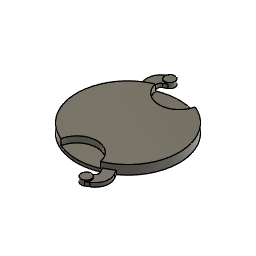
Deckbox - Key (Autodesk Fusion 360 design; units mm, degrees)
Autodesk Fusion 360 part; units mm, degrees
sketch "Sketch1" plane through (0, 0, 0) normal (0, 1, 0) x (1, 0, 0)
  circle A0 centre (0, 0) radius 25.4
  line L0 (19.5918, -28.934) -> (-15.2617, 31.434)
  line L1 (-19.5918, 28.934) -> (15.2617, -31.434)
  line L2 (0, -25.4) -> (0, 25.4) construction
  line L3 (0, 0) -> (25.4, 0) construction
  line L4 (-19.5918, 28.934) -> (-15.2617, 31.434)
  line L5 (15.2617, -31.434) -> (19.5918, -28.934)
  line L6 (17.4268, -30.184) -> (-17.4268, 30.184) construction
  line L7 (-2.1651, -1.25) -> (2.1651, 1.25) construction
  line L8 (19.5918, -28.934) -> (11.7976, -33.434)
  line L9 (11.7976, -33.434) -> (9.2976, -29.1039)
  line L10 (9.2976, -29.1039) -> (17.0918, -24.6039)
  line L11 (17.0918, -24.6039) -> (19.5918, -28.934)
  circle A1 centre (10.5476, -31.269) radius 2.5
  circle A2 centre (0, 0) radius 35.5
  line L12 (-19.5918, 28.934) -> (-17.0918, 24.6039)
  line L13 (-17.0918, 24.6039) -> (-9.2976, 29.1039)
  line L14 (-9.2976, 29.1039) -> (-11.7976, 33.434)
  line L15 (-11.7976, 33.434) -> (-19.5918, 28.934)
  circle A3 centre (-10.5476, 31.269) radius 2.5
  point P0 (-12.5, 21.6506)
  point P1 (12.5, -21.6506)
  dimension "d1" = 50.8
  dimension "d42" = 5
  dimension "d45" = 5
  dimension "d46" = 71
  dimension "d47" = 60
  dimension "d48" = 4
  dimension "d51" = 5
  constraint coincident A0.centre L3.start
  constraint coincident A0 L2.start
  constraint coincident A0 L2.end
  constraint coincident A0.centre L2
  constraint coincident A0 L3.end
  constraint horizontal L3
  constraint perpendicular L0 L4
  constraint perpendicular L0 L5
  constraint perpendicular L1 L4
  constraint midpoint L5 L6.start
  constraint midpoint L4 L6.end
  constraint perpendicular L4 L6
  constraint midpoint L1 L7.start
  constraint midpoint L0 L7.end
  constraint midpoint L6 A0.centre
  constraint perpendicular L8 L9
  constraint parallel L8 L10
  constraint parallel L9 L11
  constraint perpendicular L0 L8
  constraint midpoint L9 A1.centre
  constraint tangent L10 A1
  constraint concentric A0 A2
  constraint tangent A1 A2
  constraint perpendicular L12 L13
  constraint parallel L12 L14
  constraint parallel L13 L15
  constraint coincident L1 L12.end
  constraint midpoint L14 A3.centre
  constraint tangent L13 A3
  constraint tangent A2 A3
  measures "d1" diameter of A0
  measures "d42" distance of L0 L1
  measures "d45" diameter of A1
  measures "d46" diameter of A2 A0.centre
  measures "d47" angle of L3 L6
  measures "d48" distance of L1 A1.centre
  measures "d51" diameter of A3
extrude "Extrude1" add sketch "Sketch1" along normal blind 4.5 contours A0 L0 | A0 L0 L1 | A0 L1
extrude "Extrude2" add sketch "Sketch1" along normal blind 1.9 contours A0 L0 | A0 L0 L1 | A0 L0 L1 L13 | A0 L0 L1 L10 | A0 L1 | L0 L1 L4 L12 L13 L15 | L0 L13 L15 A3 | L0 L1 L5 L8 L10 L11 | L14 A3 | L14 A3 | L1 L8 L10 A1 | L9 A1 | L9 A1
extrude "Extrude3" add sketch "Sketch1" along normal blind 2.5 contours L14 A3 | L14 A3 | L9 A1 | L9 A1
sketch "Sketch2" plane through (0, 4.5, 0) normal (0, 1, 0) x (-1, 0, 0)
  circle A0 centre (0, 0) radius 25.4
  circle A1 centre (0, -25.4) radius 10
  circle A2 centre (0, 25.4) radius 10
  line L0 (0, -25.4) -> (0, 25.4) construction
  dimension "d18" = 20
  dimension "d19" = 20
  constraint coincident A0 A1.centre
  constraint coincident A0 A2.centre
  constraint coincident A1.centre L0.start
  constraint coincident A2.centre L0.end
  constraint coincident A0.centre L0
  constraint vertical L0
  measures "d18" diameter of A1
  measures "d19" diameter of A2
extrude "Extrude4" cut sketch "Sketch2" against normal blind 3 contours A0 A2 | A0 A1 picked at (-1.832, 22.0709) picked at (1.832, -22.0709)
fillet "Fillet6" radius 2 2 edges at (12.7617, 0.95, 27.1039) (-12.7617, 0.95, -27.1039)
fillet "Fillet7" radius 7 2 edges at (19.5918, 0.95, 28.934) (-19.5918, 0.95, -28.934)
named bodies: "Deckbox - Key"
